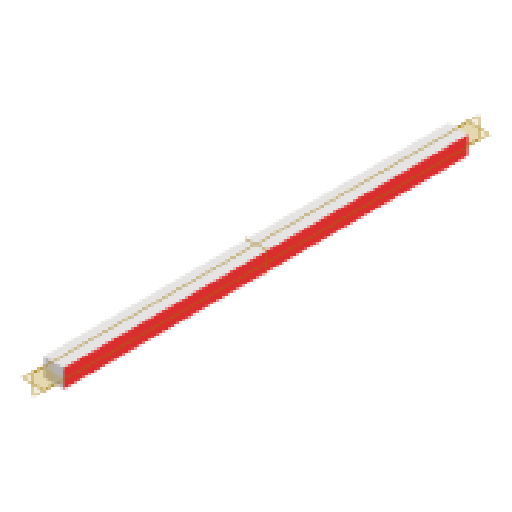
# Autodesk Inventor part: Проставка для боковых фанер
Saved by Autodesk Inventor 2023.2 (Build 272271030, 271C)
## iProperties
Created: 2025-04-24
Part Number: Проставка для боковых фанер
Material: Типовые
Document SubType Name: Modeling
Designer: Коноваленко
Density: 1 g/cm^3
Appearance: По умолчанию
Author: Коноваленко
Autodesk Inventor part; units mm, degrees
sketch "Эскиз1" plane through (0, 0, 0) normal (1, 0, 0) x (0, 1, 0)
  line L0 (-10, -220) -> (10, -220)
  line L1 (10, -220) -> (10, 220)
  line L2 (10, 220) -> (-10, 220)
  line L3 (-10, 220) -> (-10, -220)
  line L4 (-10, -220) -> (10, 220) construction
  line L5 (10, -220) -> (-10, 220) construction
  line L6 (0, 417.2) -> (0, -326.2) construction
  line L7 (-14, 0) -> (14, 0) construction
  line L8 (-10, 311) -> (-10, 220) projected
  line L9 (10, 220) -> (-10, 311)
  point P0 (0, 0)
  point P1 (0, 0)
  constraints: 14 end point, 3 midpoint, 2 parallel, 1 horizontal, 1 perpendicular, 1 point on line
extrude "Выдавливание1" add sketch "Эскиз1" along normal mid plane 22 contours L3 L2 L1 L0
